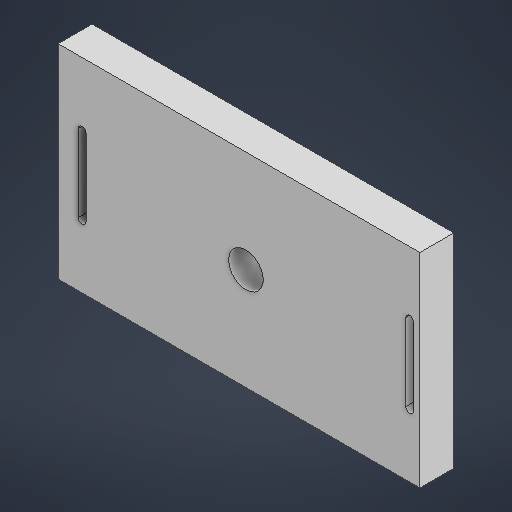
# Autodesk Inventor part: base
Saved by Autodesk Inventor 2026.2 (Build 302298010, 298A)
## iProperties
Created: 2026-03-02
Part Number: base
Material: Generic
Document SubType Name: Modeling
Designer: shahd
Density: 1 g/cm^3
Appearance: Default
Author: shahd
Autodesk Inventor part; units mm, degrees
ref_plane "YZ Plane" through (0, 0, 0) normal (1, 0, 0) x (0, 1, 0)
ref_plane "XZ Plane" through (0, 0, 0) normal (0, 1, 0) x (-1, 0, 0)
ref_plane "XY Plane" through (0, 0, 0) normal (0, 0, 1) x (1, 0, 0)
sketch "Sketch1" plane through (0, 0, 0) normal (0, 0, 1) x (1, 0, 0)
  line L0 (0, 0) -> (150, 0)
  line L1 (150, 0) -> (150, 60)
  line L2 (150, 60) -> (0, 60)
  line L3 (0, 60) -> (0, 0)
  dimension "d1" = 60
  constraints: 8 end point, 2 parallel, 1 horizontal, 1 perpendicular, 1 other
  measures "d1" distance of L0.end L1.end
extrude "Extrusion1" add sketch "Sketch1" along normal blind 10
sketch "Sketch2" plane through (0, 0, 0) normal (0, 0, -1) x (-1, 0, 0)
  line L0 (-150, 60) -> (0, 60) projected
  line L1 (0, 0) -> (-150, 0) projected
  circle A0 centre (-98.8, 30) radius 5.1
  dimension "d5" = 10.2
  dimension "d6" = 30
  dimension "d20" = 98.8
  constraints: 1 centre point
  measures "d5" diameter of A0
  measures "d6" distance from line of A0.centre L1
  measures "d20" horizontal distance of L1.start A0.centre
extrude "Extrusion2" cut sketch "Sketch2" against normal blind 10
sketch "Sketch3" plane through (0, 0, 0) normal (0, 0, -1) x (-1, 0, 0)
  line L0 (-147, 18.65) -> (-147, 41.35) construction
  line L1 (-145.85, 18.65) -> (-145.85, 41.35)
  line L2 (-148.15, 41.35) -> (-148.15, 18.65)
  arc A0 (-148.15, 18.65) -> (-145.85, 18.65) centre (-147, 18.65) ccw
  arc A1 (-145.85, 41.35) -> (-148.15, 41.35) centre (-147, 41.35) ccw
  line L3 (0, 0) -> (-150, 0) projected
  circle A2 centre (-98.8, 30) radius 5.1 projected
  circle A3 centre (-98.8, 30) radius 5.1 projected
  line L4 (-150, 0) -> (-150, 60) projected
  line L5 (-150, 60) -> (0, 60) projected
  line L6 (0, 60) -> (0, 0) projected
  line L7 (0, 0) -> (-150, 0) projected
  line L8 (-50.6, 18.65) -> (-50.6, 41.35) construction
  line L9 (-49.45, 18.65) -> (-49.45, 41.35)
  line L10 (-51.75, 41.35) -> (-51.75, 18.65)
  arc A4 (-51.75, 18.65) -> (-49.45, 18.65) centre (-50.6, 18.65) ccw
  arc A5 (-49.45, 41.35) -> (-51.75, 41.35) centre (-50.6, 41.35) ccw
  point P0 (-147, 30)
  point P1 (-147, 42.5)
  point P2 (-147, 17.5)
  point P3 (-50.6, 30)
  point P4 (-50.6, 42.5)
  point P5 (-50.6, 17.5)
  dimension "d10" = 2.3
  dimension "d12" = 25
  dimension "d17" = 3
  dimension "d27" = 2.3
  dimension "d28" = 25
  dimension "d29" = 48.2
  constraints: 16 end point, 12 point on circle, 8 tangent, 4 centre point, 3 horizontal alignment, 2 midpoint, 2 parallel, 1 coincident, 1 vertical
  measures "d10" diameter of A1
  measures "d12" distance of point (-147, 42.5) point (-147, 17.5)
  measures "d17" horizontal distance of L3.end point (-147, 30)
  measures "d27" diameter of A5
  measures "d28" distance of point (-50.6, 42.5) point (-50.6, 17.5)
  measures "d29" distance of point (-50.6, 30) A3.centre
extrude "Extrusion3" cut sketch "Sketch3" against normal blind 10 contours A0 L2 A1 L1 | A4 L10 A5 L9
sketch "Sketch4" plane through (0, 0, 10) normal (0, 0, 1) x (1, 0, 0)
  line L0 (0, 60) -> (0, 0) projected
  line L1 (150, 60) -> (0, 60) projected
  line L2 (0, 0) -> (43.5504, 0)
  line L3 (43.5504, 0) -> (43.5504, 60)
  line L4 (43.5504, 60) -> (0, 60)
  line L5 (0, 60) -> (0, 0)
  constraints: 8 end point, 2 parallel, 1 horizontal, 1 perpendicular, 1 point on line
extrude "Extrusion4" cut sketch "Sketch4" against normal through all
body "Solid1"
